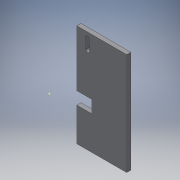
# Autodesk Inventor part: XMotorMount
Saved by Autodesk Inventor 2019 (Build 230136000, 136)
## iProperties
Created: 2018-10-14
Part Number: XMotorMount
Material: Generic
Document SubType Name: Modeling
Designer: LillaHunden
Density: 1 g/cm^3
Appearance: Default
Author: LillaHunden
Autodesk Inventor part; units mm, degrees
ref_plane "YZ Plane" through (0, 0, 0) normal (1, 0, 0) x (0, 1, 0)
ref_plane "XZ Plane" through (0, 0, 0) normal (0, 1, 0) x (-1, 0, 0)
ref_plane "XY Plane" through (0, 0, 0) normal (0, 0, 1) x (1, 0, 0)
sketch "Sketch1" plane through (0, 0, 0) normal (0, 0, 1) x (1, 0, 0)
  line L0 (112.0815, -42.6698) -> (40.0716, -42.6698)
  line L1 (40.0716, -42.6698) -> (40.0716, 105.1384)
  line L2 (40.0716, 105.1384) -> (112.0815, 105.1384)
  line L3 (112.0815, 105.1384) -> (112.0815, -42.6698)
  point P0 (0, 0)
  constraints: 8 end point, 2 parallel, 1 horizontal, 1 perpendicular
extrude "Extrusion1" add sketch "Sketch1" along normal blind 6
sketch "Sketch2" plane through (0, 0, 6) normal (0, 0, 1) x (1, 0, 0)
  point P0 (0, 0)
sketch "Sketch3" plane through (0, 0, 6) normal (0, 0, 1) x (1, 0, 0)
  circle A0 centre (45.9019, 8.4802) radius 3.25 construction
  circle A1 centre (55.0716, 8.4786) radius 3.25 construction
  circle A2 centre (55.0716, 1.1818) radius 3.25 construction
  circle A3 centre (45.9019, 1.1802) radius 3.25 construction
  line L0 (-13.5113, -2.6698) -> (60.0076, -2.6698) construction
  line L1 (60.0076, -2.6698) -> (60.0076, 12.3302) construction
  line L2 (-13.5113, 12.3302) -> (60.0076, 12.3302) construction
  line L3 (-13.5113, -2.6698) -> (-13.5113, 12.3302) construction
  line L4 (40.0716, 105.1384) -> (40.0716, -42.6698) projected
  line L5 (40.0716, 13.8302) -> (61.5076, 13.8302)
  line L6 (61.5076, 13.8302) -> (61.5076, -4.1698)
  line L7 (61.5076, -4.1698) -> (40.0716, -4.1698)
  line L8 (40.0716, -4.1698) -> (40.0716, 13.8302)
  point P0 (0, 0)
  dimension "d2" = 1.5
  dimension "d3" = 1.5
  dimension "d4" = 1.5
  constraints: 8 end point, 2 parallel, 1 horizontal, 1 perpendicular, 1 point on line
  measures "d2" distance between parallel lines of L0 L7
  measures "d3" distance between parallel lines of L5 L2
  measures "d4" distance between parallel lines of L6 L1
extrude "Extrusion2" cut sketch "Sketch3" against normal through all
sketch "Sketch4" plane through (0, 0, 6) normal (0, 0, 1) x (1, 0, 0)
  circle A0 centre (102.6515, 97.6673) radius 2.8 construction
  circle A1 centre (55.5115, 97.6673) radius 2.8 construction
  circle A2 centre (55.5115, 50.5273) radius 2.8 construction
  circle A3 centre (102.6515, 50.5273) radius 2.8 construction
  line L0 (55.5115, 97.6673) -> (55.5115, 87.6673) construction
  line L1 (52.7115, 97.6673) -> (52.7115, 87.6673)
  line L2 (58.3115, 87.6673) -> (58.3115, 97.6673)
  arc A4 (58.3115, 97.6673) -> (52.7115, 97.6673) centre (55.5115, 97.6673) ccw
  arc A5 (52.7115, 87.6673) -> (58.3115, 87.6673) centre (55.5115, 87.6673) ccw
  point P0 (0, 0)
  point P1 (55.5115, 92.6673)
  dimension "d7" = 10
  constraints: 8 end point, 4 point on circle, 4 tangent, 2 centre point, 1 midpoint, 1 parallel, 1 vertical
  measures "d7" distance of L0.start L0.end
extrude "Extrusion3" cut sketch "Sketch4" against normal through all
pattern_linear "Rectangular Pattern1" count 2 spacing 47.14 along (1, 0, 0) count 2 spacing 47.14 along (0, -1, 0) of "Extrusion3"
sketch "Sketch5" plane through (0, 0, 0) normal (0, 0, -1) x (-1, 0, 0)
  circle A0 centre (-79.0815, 74.3922) radius 19.5 construction
  line L0 (-79.0815, 74.3922) -> (-79.0815, 64.3922) construction
  line L1 (-99.0815, 74.3922) -> (-99.0815, 64.3922)
  line L2 (-59.0815, 64.3922) -> (-59.0815, 74.3922)
  arc A1 (-59.0815, 74.3922) -> (-99.0815, 74.3922) centre (-79.0815, 74.3922) ccw
  arc A2 (-99.0815, 64.3922) -> (-59.0815, 64.3922) centre (-79.0815, 64.3922) ccw
  point P0 (0, 0)
  point P1 (-79.0815, 69.3922)
  dimension "d16" = 10
  dimension "d17" = 40
  constraints: 8 end point, 4 point on circle, 4 tangent, 2 centre point, 1 midpoint, 1 parallel, 1 vertical
  measures "d16" distance of L0.start L0.end
  measures "d17" diameter of A2
extrude "Extrusion4" cut sketch "Sketch5" against normal blind 2
sketch "Sketch6" plane through (0, 0, 6) normal (0, 0, 1) x (1, 0, 0)
  arc A0 (80.8837, 71.7722) -> (77.2793, 71.7722) centre (79.0815, 74.3922) ccw construction
  line L0 (79.0815, 74.3922) -> (79.0815, 64.3922) construction
  line L1 (75.5815, 74.3922) -> (75.5815, 64.3922)
  line L2 (82.5815, 64.3922) -> (82.5815, 74.3922)
  arc A1 (82.5815, 74.3922) -> (75.5815, 74.3922) centre (79.0815, 74.3922) ccw
  arc A2 (75.5815, 64.3922) -> (82.5815, 64.3922) centre (79.0815, 64.3922) ccw
  line L3 (79.0815, 74.3922) -> (89.0815, 74.3922) construction
  point P0 (0, 0)
  point P1 (79.0815, 69.3922)
  dimension "d20" = 10
  dimension "d21" = 90
  dimension "d22" = 7
  constraints: 10 end point, 4 point on circle, 4 tangent, 2 centre point, 1 horizontal, 1 midpoint, 1 parallel, 1 perpendicular, 1 vertical
  measures "d20" distance of L0.start L0.end
  measures "d21" angle of L0 L3
  measures "d22" diameter of A2
extrude "Extrusion5" cut sketch "Sketch6" against normal through all
body "Solid1"
